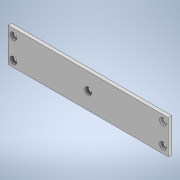
# Autodesk Inventor part: Пластинка шасси
Saved by Autodesk Inventor 2022 (Build 260153000, 153)
## iProperties
Created: 2022-07-09
Part Number: Пластинка шасси
Material: Типовые
Document SubType Name: Modeling
Designer: Константин
Density: 1 g/cm^3
Appearance: По умолчанию
Author: Константин
Autodesk Inventor part; units mm, degrees
ref_plane "YZ Plane" through (0, 0, 0) normal (1, 0, 0) x (0, 1, 0)
ref_plane "XZ Plane" through (0, 0, 0) normal (0, 1, 0) x (-1, 0, 0)
ref_plane "XY Plane" through (0, 0, 0) normal (0, 0, 1) x (1, 0, 0)
sketch "Эскиз1" plane through (0, 0, 0) normal (0, 0, 1) x (1, 0, 0)
  line L0 (-43.165, 23.4115) -> (48.835, 23.4115)
  line L1 (48.835, 23.4115) -> (48.835, 3.9115)
  line L2 (48.835, 3.9115) -> (-43.165, 3.9115)
  line L3 (-43.165, 3.9115) -> (-43.165, 23.4115)
  point P0 (0, 0)
  dimension "d0" = 92
  dimension "d1" = 19.5
  constraints: 8 end point, 3 perpendicular, 1 horizontal
  measures "d0" distance of L0.start L0.end
  measures "d1" distance of L2.end L0.start
extrude "Выдавливание1" add sketch "Эскиз1" along normal blind 2
sketch "Эскиз2" plane through (0, 0, 2) normal (0, 0, 1) x (1, 0, 0)
  circle A0 centre (-40.165, 7.4115) radius 2
  line L0 (-43.165, 23.4115) -> (-43.165, 3.9115) projected
  line L1 (-43.165, 3.9115) -> (48.835, 3.9115) projected
  circle A1 centre (-40.165, 19.4115) radius 2
  line L2 (48.835, 23.4115) -> (-43.165, 23.4115) projected
  circle A2 centre (45.835, 19.9115) radius 2
  line L3 (48.835, 3.9115) -> (48.835, 23.4115) projected
  circle A3 centre (45.835, 7.9115) radius 2
  circle A4 centre (2.835, 13.6615) radius 2
  point P0 (0, 0)
  dimension "d4" = 1
  dimension "d5" = 4
  dimension "d6" = 1.5
  dimension "d7" = 4
  dimension "d8" = 1
  dimension "d9" = 2
  dimension "d10" = 4
  dimension "d11" = 1
  dimension "d12" = 1.5
  dimension "d13" = 4
  dimension "d14" = 1
  dimension "d15" = 2
  dimension "d16" = 4
  dimension "d17" = 44
  dimension "d19" = 7.75
  constraints: 5 centre point
  measures "d4" distance edge to line of A0 L0
  measures "d5" diameter of A0
  measures "d6" distance edge to line of A0 L1
  measures "d7" diameter of A1
  measures "d8" distance edge to line of A1 L0
  measures "d9" distance edge to line of A1 L2
  measures "d10" diameter of A2
  measures "d11" distance edge to line of A2 L3
  measures "d12" distance edge to line of A2 L2
  measures "d13" diameter of A3
  measures "d14" distance edge to line of A3 L3
  measures "d15" distance edge to line of A3 L1
  measures "d16" diameter of A4
  measures "d17" distance edge to line of A4 L0
  measures "d19" distance edge to line of A4 L2
extrude "Выдавливание2" cut sketch "Эскиз2" against normal through all contours A0 | A1 | A2 | A3 | A4
